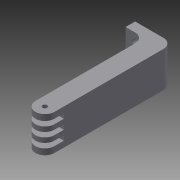
# Autodesk Inventor part: WebcamArm
Saved by Autodesk Inventor 2015 (Build 190159000, 159)
## iProperties
Created: 2015-05-12
Part Number: WebcamArm
Material: Generic
Document SubType Name: Modeling
Designer: Kurtis
Density: 1 g/cm^3
Appearance: Default
Author: Kurtis
Autodesk Inventor part; units mm, degrees
ref_plane "YZ Plane" through (0, 0, 0) normal (1, 0, 0) x (0, 1, 0)
ref_plane "XZ Plane" through (0, 0, 0) normal (0, 1, 0) x (-1, 0, 0)
ref_plane "XY Plane" through (0, 0, 0) normal (0, 0, 1) x (1, 0, 0)
sketch "Sketch1" plane through (0, 0, 0) normal (0, 0, 1) x (1, 0, 0)
  line L0 (0, 0) -> (0, 50)
  line L1 (0, 50) -> (-8, 50)
  line L2 (0, 0) -> (8, 0)
  line L3 (8, 0) -> (8, 54)
  line L4 (8, 54) -> (-8, 54)
  line L5 (8, 54) -> (-8, 54)
  line L6 (-8, 54) -> (-8, 50)
  dimension "d0" = 50
  dimension "d3" = 8
  dimension "d7" = 54
  dimension "d28" = 16
  constraints: 14 end point, 4 perpendicular, 1 horizontal, 1 vertical
  measures "d0" distance of L0.start L0.end
  measures "d3" distance of L0.start L2.end
  measures "d7" distance between parallel lines of L5 L2
  measures "d28" distance between parallel lines of L3 L6
extrude "Extrusion1" add sketch "Sketch1" along normal blind 15
sketch "Sketch2" plane through (-8, 54, 0) normal (0, 1, 0) x (1, 0, 0)
  line L0 (16, 0) -> (0, 0) construction
  line L1 (1.2766, 0) -> (1.2766, -15) construction
  line L2 (16, -15) -> (0, -15) construction
  line L3 (1.2766, 0) -> (1.2766, -2.75) construction
  line L4 (1.2766, -15) -> (1.2766, -12.25) construction
  line L5 (1.2766, 0) -> (1.2766, -3.5) construction
  line L6 (1.2766, -15) -> (1.2766, -11.5) construction
  line L7 (8, 0) -> (0, 0) construction
  line L8 (0, 0) -> (0, -15) construction
  line L9 (4, 0) -> (4, -15) construction
  line L10 (4, -15) -> (4, -11.5) construction
  line L11 (4, 0) -> (4, -3.5) construction
  circle A0 centre (4, -3.5) radius 1.5
  circle A1 centre (4, -11.5) radius 1.5
  dimension "d12" = 3.5
  dimension "d13" = 3.5
  dimension "d29" = 3.5
  dimension "d30" = 3.5
  dimension "d31" = 3
  dimension "d32" = 3
  constraints: 18 end point, 8 point on line, 2 centre point, 2 coincident, 2 perpendicular, 1 midpoint
  measures "d12" distance of L1.start L5.end
  measures "d13" distance of L1.end L6.end
  measures "d29" distance of L9.end L10.end
  measures "d30" distance of L9.start L11.end
  measures "d31" diameter of A0
  measures "d32" diameter of A1
extrude "Extrusion2" cut sketch "Sketch2" against normal blind 8.75
sketch "Sketch3" plane through (8, 0, 0) normal (1, 0, 0) x (0, 0, -1)
  line L0 (0, 0) -> (-15, 0) construction
  line L1 (-7.5, 0) -> (-7.5, 8) construction
  line L2 (-7.5, 8) -> (-6.5, 8)
  line L3 (-6.5, 8) -> (-8.5, 8)
  line L4 (-8.5, 8) -> (-8.5, 0)
  line L5 (-6.5, 8) -> (-6.5, 0)
  line L6 (-6.5, 0) -> (-4.5, 0)
  line L7 (-4.5, 0) -> (-4.5, 8)
  line L8 (-4.5, 8) -> (-2.5, 8)
  line L9 (-2.5, 8) -> (-2.5, 0)
  line L10 (-8.5, 0) -> (-10.5, 0)
  line L11 (-10.5, 0) -> (-10.5, 8)
  line L12 (-10.5, 8) -> (-12.5, 8)
  line L13 (-12.5, 8) -> (-12.5, 0)
  line L14 (-2.5, 0) -> (0, 0)
  line L15 (-12.5, 0) -> (-15, 0)
  line L16 (-15, 0) -> (-15, 10)
  line L17 (-15, 50) -> (-15, 0) projected
  line L18 (-15, 10) -> (0, 10)
  line L19 (0, 50) -> (0, 0) projected
  line L20 (0, 0) -> (0, 10)
  line L21 (-15, 0) -> (0, 0)
  dimension "d18" = 8
  dimension "d19" = 1
  dimension "d20" = 2
  dimension "d21" = 2
  dimension "d22" = 2
  dimension "d23" = 2
  dimension "d24" = 2
  dimension "d25" = 10
  constraints: 38 end point, 8 perpendicular, 5 point on line, 3 vertical, 2 horizontal, 1 parallel, 8 other
  measures "d18" distance of L1.start L1.end
  measures "d19" distance of L1.end L2.end
  measures "d20" distance of L2.end L3.end
  measures "d21" distance of L5.end L6.end
  measures "d22" distance of L7.end L8.end
  measures "d23" distance of L4.end L10.end
  measures "d24" distance of L11.end L12.end
  measures "d25" distance of L15.end L16.end
extrude "Extrusion3" cut sketch "Sketch3" against normal blind 10.25 contours L2 L5 L21 L4 L3 | L7 L8 L9 L21 | L21 L13 L12 L11
fillet "Fillet1" radius 4 8 edges at (8, 0, 1.25) (8, 0, 5.5) (8, 0, 9.5) (8, 0, 13.75) (0, 0, 13.75) (0, 0, 9.5) (0, 0, 5.5) (0, 0, 1.25)
sketch "Sketch4" plane through (0, 0, 15) normal (0, 0, 1) x (1, 0, 0)
  line L0 (0, 4) -> (8, 4) construction
  circle A0 centre (4, 4) radius 1
  point P0 (0, 0)
  dimension "d34" = 2
  constraints: 2 end point, 1 centre point, 1 midpoint
  measures "d34" diameter of A0
extrude "Extrusion4" cut sketch "Sketch4" against normal blind 21
fillet "Fillet2" radius 4 2 edges at (8, 54, 7.5) (0, 50, 7.5)
body "Solid1"
